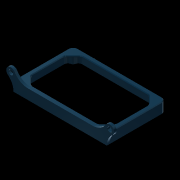
# Autodesk Inventor part: 3d_DAA - Glass mount
Saved by Autodesk Inventor 2018 (Build 220112000, 112)
## iProperties
Category: 0
Created: 2024-09-02
Part Number: 3d_DAA - Glass mount
Material: Aluminium 6061-T6
Document SubType Name: Modeling
Designer: cda1
Density: 2.7 g/cm^3
Appearance: Pantone 2965 U - Anodized
Mass: 11.5373 g
Surface Area: 55.5304 cm^2
Volume: 4.27308 cm^3
Manufacturer-1: {"Link": "", "Name": "SHENZHEN JINYIHE PROTOTYPE TECHNOLOGIES CO., LTD (JYH)", "PartNumber": "3d_DAA - Glass mount", "partner_id": false}
Manufacturer-2: {"Link": "", "Name": "QICHUANG MOLD CO., LTD", "PartNumber": "3d_DAA - Glass mount", "partner_id": false}
Manufacturer-3: {"Link": "", "Name": "SUNPE LIMITED", "PartNumber": "3d_DAA - Glass mount", "partner_id": false}
Manufacturer-4: {"Link": "", "Name": "", "PartNumber": "", "partner_id": false}
Manufacturer-5: {"Link": "", "Name": "", "PartNumber": "", "partner_id": false}
Provider-1: {"Link": "", "Name": "", "PartNumber": "", "partner_id": false}
Provider-2: {"Link": "", "Name": "", "PartNumber": "", "partner_id": false}
Provider-3: {"Link": "", "Name": "", "PartNumber": "", "partner_id": false}
Provider-4: {"Link": "", "Name": "", "PartNumber": "", "partner_id": false}
Provider-5: {"Link": "", "Name": "", "PartNumber": "", "partner_id": false}
odoo_id: 17985
odoo_internal_code: P010350
odoo_model: product.product
odoo_x2o_application_version: 12.0.4.10
odoo_d2o_version: 12.0.1.4.34
Author: cda1
Comments: DIN-2768-1-fine
Autodesk Inventor part; units mm, degrees
ref_plane "YZ Plane" through (0, 0, 0) normal (1, 0, 0) x (0, 1, 0)
ref_plane "XZ Plane" through (0, 0, 0) normal (0, 1, 0) x (-1, 0, 0)
ref_plane "XY Plane" through (0, 0, 0) normal (0, 0, 1) x (1, 0, 0)
sketch "Boceto1" plane through (0, 0, 0) normal (0, 0, 1) x (1, 0, 0)
  line L0 (-34, 19) -> (-34, -19)
  arc A0 (-34, -19) -> (-32, -21) centre (-32, -19) ccw
  line L1 (-32, -21) -> (32, -21)
  arc A1 (32, -21) -> (34, -19) centre (32, -19) ccw
  line L2 (34, -19) -> (34, 19)
  arc A2 (34, 19) -> (32, 21) centre (32, 19) ccw
  line L3 (32, 21) -> (-32, 21)
  arc A3 (-32, 21) -> (-34, 19) centre (-32, 19) ccw
  line L4 (-32, 23) -> (32, 23)
  line L5 (36, 19) -> (36, -23)
  line L6 (36, -23) -> (-36, -23)
  line L7 (-36, -23) -> (-36, 19)
  arc A4 (-32, 23) -> (-36, 19) centre (-32, 19) ccw
  arc A5 (36, 19) -> (32, 23) centre (32, 19) ccw
  point P0 (0, 0)
  dimension "d1" = 2
  dimension "d3" = 2
  dimension "d4" = 4
  dimension "d97" = 2
  dimension "d102" = 2
  dimension "d103" = 34
  dimension "d104" = 34
  dimension "d105" = 21
  dimension "d107" = 21
  dimension "d108" = 2
  dimension "d109" = 2
  dimension "d110" = 2
  dimension "d111" = 2
  constraints: 16 end point, 12 point on circle, 12 tangent, 6 centre point, 2 parallel, 1 equal radius, 1 horizontal, 1 perpendicular
  measures "d1" distance between parallel lines of L4 L3
  measures "d3" distance between parallel lines of L6 L1
  measures "d4" radius of A4
  measures "d97" distance between parallel lines of L2 L5
  measures "d102" distance between parallel lines of L7 L0
  measures "d103" distance from line of L2 point (0, 0)
  measures "d104" distance from line of L0 point (0, 0)
  measures "d105" distance from line of L3 point (0, 0)
  measures "d107" distance from line of L1 point (0, 0)
  measures "d108" radius of A1
  measures "d109" radius of A0
  measures "d110" radius of A3
  measures "d111" radius of A2
extrude "Extrusión1" add sketch "Boceto1" along normal blind 7
sketch "Boceto2" plane through (0, 0, 0) normal (0, 0, -1) x (-1, 0, 0)
  arc A0 (-32, 23) -> (-36, 19) centre (-32, 19) ccw projected
  line L0 (-32, 23) -> (32, 23) projected
  arc A1 (36, 19) -> (32, 23) centre (32, 19) ccw projected
  line L1 (36, 19) -> (36, -23) projected
  line L2 (36, -23) -> (-36, -23) projected
  line L3 (-36, -23) -> (-36, 19) projected
  arc A2 (-32, 22) -> (-35, 19) centre (-32, 19) ccw
  line L4 (-32, 22) -> (32, 22)
  arc A3 (35, 19) -> (32, 22) centre (32, 19) ccw
  line L5 (35, 19) -> (35, -22)
  line L6 (35, -22) -> (-35, -22)
  line L7 (-35, -22) -> (-35, 19)
  arc A4 (-32, 21) -> (-34, 19) centre (-32, 19) ccw projected
  line L8 (-32, 21) -> (32, 21) projected
  line L9 (-34, -19) -> (-34, 19) projected
  line L10 (34, 19) -> (34, -19) projected
  arc A5 (34, 19) -> (32, 21) centre (32, 19) ccw projected
  arc A6 (32, -21) -> (34, -19) centre (32, -19) ccw projected
  line L11 (32, -21) -> (-32, -21) projected
  arc A7 (-34, -19) -> (-32, -21) centre (-32, -19) ccw projected
  point P0 (0, 0)
  dimension "d7" = 1
  constraints: 8 end point, 4 point on circle, 2 centre point, 5 other
  measures "d7" radial gap between concentric circles of A0 A2
sketch "Boceto4" plane through (0, 0, 7) normal (0, 0, 1) x (1, 0, 0)
  arc A0 (-32, 21) -> (-34, 19) centre (-32, 19) ccw construction
  line L0 (-32, 21) -> (32, 21) construction
  arc A1 (34, 19) -> (32, 21) centre (32, 19) ccw construction
  line L1 (34, 19) -> (34, -19) construction
  arc A2 (32, -21) -> (34, -19) centre (32, -19) ccw construction
  line L2 (32, -21) -> (-32, -21) construction
  arc A3 (-34, -19) -> (-32, -21) centre (-32, -19) ccw construction
  line L3 (-34, -19) -> (-34, 19) construction
  line L4 (36, -23) -> (36, 19) projected
  arc A4 (36, 19) -> (32, 23) centre (32, 19) ccw projected
  line L5 (32, 23) -> (-32, 23) projected
  arc A5 (-32, 23) -> (-36, 19) centre (-32, 19) ccw projected
  line L6 (-36, 19) -> (-36, -23) projected
  line L7 (-36, -23) -> (36, -23) projected
  line L8 (35, -23) -> (35, 19) projected
  line L9 (32.5, 19.5) -> (-32.5, 19.5)
  line L10 (-32.5, 19.5) -> (-32.5, -19.5)
  line L11 (-32.5, -19.5) -> (32.5, -19.5)
  line L12 (32.5, -19.5) -> (32.5, 19.5)
  arc A6 (-26, 19.5) -> (-32.5, 13) centre (-26, 13) ccw
  arc A7 (32.5, 13) -> (26, 19.5) centre (26, 13) ccw
  arc A8 (26, -19.5) -> (32.5, -13) centre (26, -13) ccw
  arc A9 (-32.5, -13) -> (-26, -19.5) centre (-26, -13) ccw
  line L13 (32.5, 13) -> (26, 19.5)
  line L14 (-26, 19.5) -> (-32.5, 13)
  line L15 (-32.5, -13) -> (-26, -19.5)
  line L16 (32.5, -13) -> (26, -19.5)
  dimension "d37" = 13
  dimension "d38" = 13
  dimension "d39" = 13
  dimension "d40" = 13
  dimension "d98" = 1.5
  dimension "d99" = 3.5
  dimension "d100" = 3.5
  dimension "d101" = 1.5
  constraints: 16 end point, 9 point on line, 8 point on circle, 8 tangent, 4 centre point, 1 perpendicular
  measures "d37" diameter of A6
  measures "d38" diameter of A7
  measures "d39" diameter of A8
  measures "d40" diameter of A9
  measures "d98" distance between parallel lines of L0 L9
  measures "d99" distance between parallel lines of L12 L4
  measures "d100" distance between parallel lines of L6 L10
  measures "d101" distance between parallel lines of L2 L11
extrude "Extrusión4" add sketch "Boceto4" along normal blind 1 contours L7 L6 A5 L5 A4 L4 | L12 A7 L9 | A7 L13 | A6 L10 L9 | L14 A6 | L12 L11 A8 | A8 L16 | A9 L11 L10 | L15 A9
sketch "Boceto5" plane through (0, 0, 7) normal (0, 0, -1) x (-1, 0, 0)
  circle A0 centre (32.3, -19.3) radius 1.5 construction
  circle A1 centre (-32.3, -19.3) radius 1.5 construction
  arc A2 (-29.8, -19.3) -> (-32.3, -16.8) centre (-32.3, -19.3) ccw
  circle A3 centre (-32.3, 19.3) radius 1.5 construction
  arc A4 (-32.3, 16.8) -> (-29.8, 19.3) centre (-32.3, 19.3) ccw
  circle A5 centre (32.3, 19.3) radius 1.5 construction
  arc A6 (29.8, 19.3) -> (32.3, 16.8) centre (32.3, 19.3) ccw
  arc A7 (34, 19) -> (32, 21) centre (32, 19) ccw construction
  line L0 (34, 19) -> (34, -19) construction
  arc A8 (32, -21) -> (34, -19) centre (32, -19) ccw construction
  line L1 (32, -21) -> (-32, -21) construction
  arc A9 (-34, -19) -> (-32, -21) centre (-32, -19) ccw construction
  line L2 (-34, -19) -> (-34, 19) construction
  arc A10 (-32, 21) -> (-34, 19) centre (-32, 19) ccw construction
  line L3 (-32, 21) -> (32, 21) construction
  line L4 (29.8, -19.3) -> (29.8, -21)
  line L5 (32.3, -16.8) -> (34, -16.8)
  arc A11 (32, -21) -> (34, -19) centre (32, -19) ccw
  line L6 (29.8, -21) -> (32, -21)
  line L7 (34, -19) -> (34, -16.8)
  arc A12 (32.3, -16.8) -> (29.8, -19.3) centre (32.3, -19.3) ccw
  line L8 (-32.3, -16.8) -> (-34, -16.8)
  line L9 (-29.8, -19.3) -> (-29.8, -21)
  arc A13 (-34, -19) -> (-32, -21) centre (-32, -19) ccw
  line L10 (-29.8, -21) -> (-32, -21)
  line L11 (-34, -16.8) -> (-34, -19)
  line L12 (-32.3, 16.8) -> (-34, 16.8)
  line L13 (-29.8, 19.3) -> (-29.8, 21)
  arc A14 (-32, 21) -> (-34, 19) centre (-32, 19) ccw
  line L14 (-34, 16.8) -> (-34, 19)
  line L15 (-29.8, 21) -> (-32, 21)
  line L16 (29.8, 19.3) -> (29.8, 21)
  line L17 (32.3, 16.8) -> (34, 16.8)
  arc A15 (34, 19) -> (32, 21) centre (32, 19) ccw
  line L18 (34, 16.8) -> (34, 19)
  line L19 (29.8, 21) -> (32, 21)
  line L20 (-32, 23) -> (32, 23) construction
  line L21 (-36, -23) -> (-36, 19) construction
  line L22 (36, -23) -> (-36, -23) construction
  line L23 (36, 19) -> (36, -23) construction
  point P0 (0, 0)
  dimension "d24" = 3
  dimension "d26" = 3
  dimension "d27" = 5
  dimension "d28" = 3
  dimension "d29" = 5
  dimension "d30" = 3
  dimension "d31" = 5
  dimension "d41" = 2.5
  dimension "d68" = 3.7
  dimension "d69" = 3.7
  dimension "d71" = 3.7
  dimension "d72" = 3.7
  constraints: 36 end point, 16 point on circle, 12 centre point, 11 tangent, 10 point on line, 8 coincident, 7 perpendicular, 2 horizontal alignment, 2 vertical alignment, 1 collinear, 1 horizontal
  measures "d24" diameter of A0
  measures "d26" diameter of A1
  measures "d27" diameter of A2
  measures "d28" diameter of A3
  measures "d29" diameter of A4
  measures "d30" diameter of A5
  measures "d31" diameter of A6
  measures "d41" radius of A12
  measures "d68" distance from line of L20 A3.centre
  measures "d69" distance from line of L21 A4.centre
  measures "d71" distance from line of L23 A5.centre
  measures "d72" distance from line of L22 A0.centre
extrude "Extrusión5" add sketch "Boceto5" along normal blind 6
fillet "Empalme1" radius 3 8 edges at (34, 16.8, 4) (29.8, 21, 4) (-29.8, 21, 4) (-34, 16.8, 4) (-34, -16.8, 4) (-29.8, -21, 4) (34, -16.8, 4) (29.8, -21, 4)
chamfer "Chaflán2" distance 0.5 angle 45 5 edges at (-34.8284, 21.8284, 8) (-36, -2, 8) (0, 23, 8) (34.8284, 21.8284, 8) (36, -2, 8)
fillet "Empalme4" radius 3 8 edges at (26, 19.5, 7.5) (32.5, 13, 7.5) (-26, 19.5, 7.5) (-32.5, 13, 7.5) (-32.5, -13, 7.5) (-26, -19.5, 7.5) (32.5, -13, 7.5) (26, -19.5, 7.5)
chamfer "Chaflán3" distance 0.5 angle 45 16 edges at (29.25, -16.25, 8) (32.2716, -12.9054, 8) (32.5, 0, 8) (32.2716, 12.9054, 8) (29.25, 16.25, 8) (25.9054, 19.2716, 8) (0, 19.5, 8) (-25.9054, 19.2716, 8) (-29.25, 16.25, 8) (-32.2716, 12.9054, 8) (-32.5, 0, 8) (-32.2716, -12.9054, 8) (-29.25, -16.25, 8) (-25.9054, -19.2716, 8) (0, -19.5, 8) (25.9054, -19.2716, 8)
extrude "Extrusión6" cut sketch "Boceto2" against normal up to surface (1 mm away) contours L4 A3 L5 L6 L7 A2
fillet "Empalme5" radius 3 2 edges at (35, -22, 0.5) (-35, -22, 0.5)
sketch "Boceto7" plane through (0, 0, 1) normal (0, 0, -1) x (-1, 0, 0)
  arc A0 (-32, 22) -> (-35, 19) centre (-32, 19) ccw construction
  arc A1 (-31.7091, 16.8708) -> (-29.8708, 18.7091) centre (-32.3, 19.3) ccw construction
  arc A2 (29.8708, 18.7091) -> (31.7091, 16.8708) centre (32.3, 19.3) ccw construction
  arc A3 (31.7091, -16.8708) -> (29.8708, -18.7091) centre (32.3, -19.3) ccw construction
  arc A4 (-29.8708, -18.7091) -> (-31.7091, -16.8708) centre (-32.3, -19.3) ccw construction
  point P0 (0, 0)
  constraints: 2 point on circle, 1 centre point
hole "Agujero2" at (32.3, 19.3, 1) at (-32.3, 19.3, 1) at (-32.3, -19.3, 1) at (32.3, -19.3, 1) direction (0, 0, 1) diameter 2.459 depth 6 thread size "M3x0.5" class "6H" standard "ISO Metric profile"
sketch "Boceto8" plane through (0, 0, 0) normal (0, 0, -1) x (-1, 0, 0)
  line L0 (-36, -23) -> (-36, 19) projected
  line L1 (36, -23) -> (-36, -23) projected
  line L2 (36, 19) -> (36, -23) projected
  arc A0 (36, 19) -> (32, 23) centre (32, 19) ccw projected
  line L3 (-32, 23) -> (32, 23) projected
  arc A1 (-32, 23) -> (-36, 19) centre (-32, 19) ccw projected
  point P0 (0, 0)
extrude "Extrusión7" cut sketch "Boceto8" against normal blind 0.2
sketch "Boceto9" plane through (-35.5, -23, 8) normal (0, -1, 0) x (1, 0, 0)
  arc A0 (75.8062, 1.3139) -> (70.5836, 5.8201) centre (73.5838, 4.0177) ccw
  circle A1 centre (73.5838, 4.0177) radius 1.7
  line L0 (-0.5, -8) -> (-0.5, -0.5) construction
  line L1 (71.5, -8) -> (71.5, -0.5) construction
  line L2 (71.5, -7.8) -> (73.5838, 4.0177) construction
  line L3 (71.5, -7.8) -> (83.5, -7.8) construction
  line L4 (-0.5, -8) -> (-0.5, -0.5) construction
  line L5 (-0.5, -7.8) -> (11.5, -7.8) construction
  line L6 (-0.5, -7.8) -> (71.5, -7.8) projected
  arc A2 (75.8062, 1.3139) -> (71.5, -7.8) centre (83.2976, -7.8) ccw
  line L7 (0, 0) -> (71, 0) construction
  arc A3 (60.2972, 0) -> (70.5836, 5.8201) centre (60.2972, 12) ccw
  line L8 (60.2972, 0) -> (71, 0)
  line L9 (60.2574, 0) -> (10.7426, 0) projected
  line L10 (71, 0) -> (71.5, -0.5)
  line L11 (71.5, -0.5) -> (71.5, -7.8)
  point P0 (35.5, -8)
  dimension "d87" = 7
  dimension "d88" = 3.4
  dimension "d89" = 80
  dimension "d91" = 12
  dimension "d94" = 12
  constraints: 13 end point, 6 point on circle, 5 tangent, 4 centre point, 2 horizontal, 1 coincident, 1 collinear, 1 equal length, 1 perpendicular, 1 point on line
  measures "d87" diameter of A0
  measures "d88" diameter of A1
  measures "d89" angle of L3 L2
  measures "d91" distance of L2.start L2.end
  measures "d94" radius of A3
extrude "Extrusión8" add sketch "Boceto9" against normal blind 2
mirror "Simetría1" about plane through (0, 0, 0) normal (1, 0, 0) of "Extrusión8"
ref_plane "Plano de trabajo1" through (0, 0, 0) normal (1, 0, 0) x (0, 1, 0)
